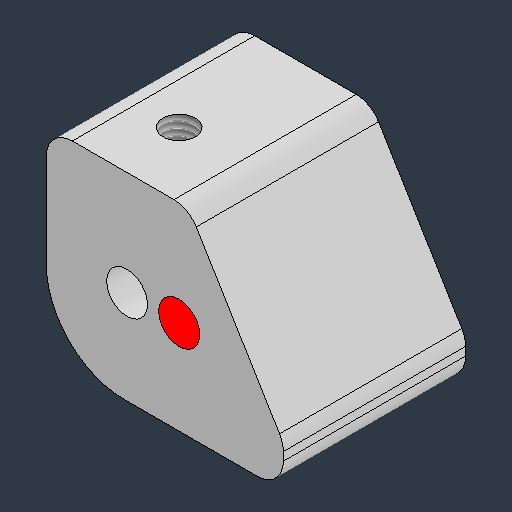
# Autodesk Inventor part: BEARING,MOUNT,SIDE,ELEVATOR
Saved by Autodesk Inventor 2024.3 (Build 283343000, 343)
## iProperties
Created: 2025-02-24
Part Number: BEARING,MOUNT,SIDE,ELEVATOR
Material: Generic
Document SubType Name: Modeling
Mfg Approved By: John.Thibert
Designer: John.Thibert
Mass: 90.3867 g
Surface Area: 38.7413 cm^2
Volume: 11.498 cm^3
Density: 7.86109 g/cm^3
Appearance: Default
ILogicPurgeVersion: 0.0.0.0
OnSaveVersion: 3.5.0.0
OnSaveAssembly: COREAutomationManager
ModelCat: Uncategorized
MaterialName: Generic
CN_MASS: 0.09
Author: John.Thibert
Autodesk Inventor part; units mm, degrees
ref_plane "YZ Plane" through (0, 0, 0) normal (1, 0, 0) x (0, 1, 0)
ref_plane "XZ Plane" through (0, 0, 0) normal (0, 1, 0) x (-1, 0, 0)
ref_plane "XY Plane" through (0, 0, 0) normal (0, 0, 1) x (1, 0, 0)
sketch "Sketch1" plane through (0, 0, 0) normal (0, 0, 1) x (1, 0, 0)
  arc A0 (5.1615, 6.0904) -> (2.4461, 7.62) centre (2.4461, 4.445) ccw construction
  line L0 (2.4461, 7.62) -> (-28.575, 7.62) construction
  arc A1 (-28.575, 7.62) -> (-31.75, 4.445) centre (-28.575, 4.445) ccw construction
  line L1 (-31.75, 4.445) -> (-31.75, -0.344) construction
  arc A2 (-31.75, -0.344) -> (-31.6418, -1.1658) centre (-28.575, -0.344) ccw construction
  line L2 (-29.5221, -9.0768) -> (-31.6418, -1.1658) construction
  arc A3 (-29.5221, -9.0768) -> (-26.4553, -11.43) centre (-26.4553, -8.255) ccw construction
  line L3 (-26.4553, -11.43) -> (9.525, -11.43) construction
  arc A4 (9.525, -11.43) -> (12.7, -8.255) centre (9.525, -8.255) ccw
  line L4 (12.7, -8.255) -> (12.7, -7.2369)
  arc A5 (12.7, -7.2369) -> (12.2404, -5.5915) centre (9.525, -7.2369) ccw
  line L5 (5.1615, 6.0904) -> (12.2404, -5.5915) construction
  line L6 (4.7625, 12.7) -> (-16.1925, 12.7)
  line L7 (-16.1925, 12.7) -> (-16.1925, -11.43)
  line L8 (-16.1925, -11.43) -> (4.7625, -11.43)
  line L9 (4.7625, -11.43) -> (4.7625, 12.7) construction
  line L10 (4.7625, -11.43) -> (9.525, -11.43)
  line L11 (12.2404, -5.5915) -> (1.1563, 12.7)
  point P0 (0, 0)
  dimension "d0" = 20.955
  dimension "d1" = 24.13
  dimension "d2" = 4.7625
  constraints: 24 end point, 12 point on circle, 6 centre point, 4 horizontal, 2 parallel, 2 point on line, 2 vertical, 1 collinear, 1 perpendicular, 1 tangent, 26 other
  measures "d0" distance of L7.end L8.end
  measures "d1" distance of L8.end L6.start
  measures "d2" distance from line of L9 point (0, 0)
extrude "Extrusion1" add sketch "Sketch1" along normal blind 22.225
sketch "Sketch2" plane through (0, 0, 22.225) normal (0, 0, 1) x (1, 0, 0)
  circle A0 centre (0, 0) radius 2.5019 construction
  circle A1 centre (-6.35, 0) radius 2.5527 construction
  circle A2 centre (-19.05, 0) radius 2.5527 construction
  circle A3 centre (-25.4, 0) radius 2.5019 construction
  point P0 (0, 0)
  constraints: 4 centre point, 8 other
hole "Hole1" at (0, 0, 22.225) direction (0, 0, -1) diameter 5.0038 end through all clearance for "H7 - STANDARD FIT" size "5" standard "CL-DOWEL-MET"
hole "Hole2" at (-6.35, 0, 22.225) at (-19.05, 0, 22.225) direction (0, 0, -1) diameter 4.9784 end through all clearance for "Flat Head Machine Screw (82)" size "#10" standard "Ansi Unified Screw Threads"
sketch "Sketch3" plane through (-16.1925, 12.7, 0) normal (0, 1, 0) x (1, 0, 0)
  line L0 (16.1925, -14.2875) -> (8.255, -14.2875) construction
  line L1 (-46.1199, -6.35) -> (861.9301, -6.35) construction
  line L2 (0, 0) -> (0, -22.225) construction
  point P0 (16.1925, 0)
  dimension "d19" = 7.9375
  dimension "d21" = 7.9375
  dimension "d31" = 8.255
  constraints: 4 end point, 2 horizontal, 2 other
  measures "d19" distance between parallel lines of L0 L1
  measures "d21" distance of L0.start L0.end
  measures "d31" distance from line of L0.end L2
hole "Hole3" at (-7.9375, 12.7, 14.2875) direction (0, -1, 0) diameter 3.9624 depth 13.6144 tip angle 118 thread size "10-32 UNF" class "2B" standard "ANSI Unified Screw Threads"
fillet "Fillet1" radius 9.525 1 edges at (-16.1925, -11.43, 11.1125)
fillet "Fillet2" radius 3.175 2 edges at (-16.1925, 12.7, 11.1125) (1.1563, 12.7, 11.1125)
body "Solid1"
